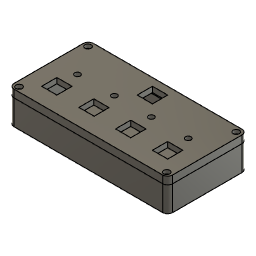
VFS5-fusion-file (Autodesk Fusion 360 design; units mm, degrees)
Autodesk Fusion 360 part; units mm, degrees
sketch "Plate" plane through (0, 0, 0) normal (0, 1, 0) x (1, 0, 0)
  line L0 (0, 0) -> (14, 0)
  line L1 (14, 0) -> (14, -14)
  line L2 (14, -14) -> (0, -14)
  line L3 (0, -14) -> (0, 0)
  line L4 (14, 0) -> (34, 0) construction
  line L5 (34, 0) -> (48, 0)
  line L6 (48, 0) -> (48, -13.6963)
  line L7 (48, -13.6963) -> (34, -13.6963)
  line L8 (34, -13.6963) -> (34, 0)
  line L9 (48, 0) -> (68, 0) construction
  line L10 (68, 0) -> (82, 0)
  line L11 (82, 0) -> (82, -14)
  line L12 (82, -14) -> (68, -14)
  line L13 (68, -14) -> (68, 0)
  line L14 (82, 0) -> (102, 0) construction
  line L15 (102, 0) -> (116, 0)
  line L16 (116, 0) -> (116, -14)
  line L17 (116, -14) -> (102, -14)
  line L18 (102, -14) -> (102, 0)
  line L19 (7, 0) -> (7, 12)
  circle A0 centre (7, 12) radius 2.55
  line L20 (41, 0) -> (41, 12)
  circle A1 centre (41, 12) radius 2.55
  line L21 (75, 0) -> (75, 12)
  circle A2 centre (75, 12) radius 2.55
  line L22 (109, 0) -> (109, 12)
  circle A3 centre (109, 12) radius 2.55
  line L23 (58, 0) -> (58, 30) construction
  line L24 (51, 23) -> (65, 23)
  line L25 (65, 23) -> (65, 37)
  line L26 (65, 37) -> (51, 37)
  line L27 (51, 37) -> (51, 23)
  line L28 (51, 23) -> (65, 37) construction
  line L29 (65, 23) -> (51, 37) construction
  line L30 (65, 37) -> (65, 42)
  line L31 (-5, -14) -> (-5, -19)
  line L32 (116, -19) -> (121, -19)
  line L33 (121, -19) -> (121, 42)
  line L34 (121, 42) -> (-5, 42)
  line L35 (-5, 42) -> (-5, -19)
  line L36 (-5, -19) -> (121, -19)
  line L37 (121, -19) -> (121, 42)
  line L38 (-5, 42) -> (-15, 42)
  line L39 (-15, 42) -> (-15, 44)
  line L40 (121, -29) -> (131, -29)
  line L41 (131, -29) -> (-15, -29)
  line L42 (-15, -29) -> (-15, 44)
  line L43 (-15, 44) -> (131, 44)
  line L44 (131, 44) -> (131, -29)
  point P0 (58, 30)
  dimension "d1" = 14
  dimension "d2" = 14
  dimension "d3" = 20
  dimension "d4" = 14
  dimension "d5" = 20
  dimension "d6" = 14
  dimension "d7" = 14
  dimension "d8" = 20
  dimension "d9" = 14
  dimension "d10" = 14
  dimension "d11" = 12
  dimension "d12" = 5.1
  dimension "d13" = 12
  dimension "d14" = 5.1
  dimension "d15" = 12
  dimension "d16" = 5.1
  dimension "d17" = 12
  dimension "d18" = 5.1
  dimension "d20" = 14
  dimension "d21" = 14
  dimension "d22" = 30
  dimension "d26" = 5
  dimension "d29" = 5
  dimension "d30" = 126
  dimension "d31" = 61
  constraint horizontal L0
  constraint vertical L1
  constraint horizontal L2
  constraint vertical L3
  constraint coincident L0.start L3.end
  constraint perpendicular L1 L4
  constraint horizontal L5
  constraint vertical L6
  constraint horizontal L7
  constraint vertical L8
  constraint perpendicular L6 L9
  constraint horizontal L10
  constraint vertical L11
  constraint horizontal L12
  constraint vertical L13
  constraint perpendicular L11 L14
  constraint horizontal L15
  constraint vertical L16
  constraint horizontal L17
  constraint vertical L18
  constraint midpoint L0 L19.start
  constraint perpendicular L0 L19
  constraint coincident L19.end A0.centre
  constraint coincident L20.end A1.centre
  constraint coincident L21.end A2.centre
  constraint coincident L22.end A3.centre
  constraint midpoint L9 L23.start
  constraint horizontal L24
  constraint perpendicular L24 L25
  constraint parallel L24 L26
  constraint parallel L25 L27
  constraint coincident L28 P0
  constraint coincident L29 P0
  constraint coincident P0 L23.end
  constraint perpendicular L26 L30
  constraint horizontal L34
  constraint vertical L35
  constraint horizontal L36
  constraint vertical L37
  constraint perpendicular L35 L38
  constraint perpendicular L38 L39
  constraint horizontal L41
  constraint vertical L42
  constraint horizontal L43
  constraint vertical L44
  measures "d1" distance of L0.start L0.end
  measures "d2" distance of L0.start L2.end
  measures "d3" distance of L0.end L4.end
  measures "d4" distance of L4.end L5.end
  measures "d5" distance of L5.end L9.end
  measures "d6" distance of L9.end L10.end
  measures "d7" distance of L9.end L12.end
  measures "d8" distance of L10.end L14.end
  measures "d9" distance of L14.end L15.end
  measures "d10" distance of L14.end L17.end
  measures "d11" distance of L19.start L19.end
  measures "d12" diameter of A0
  measures "d13" distance of L20.start L20.end
  measures "d14" diameter of A1
  measures "d15" distance of L21.start L21.end
  measures "d16" diameter of A2
  measures "d17" distance of L22.start L22.end
  measures "d18" diameter of A3
  measures "d20" distance of L25.end L26.end
  measures "d21" distance of L24.end L25.end
  measures "d22" distance of L23.start P0
  measures "d26" distance of L16.end L32.start
  measures "d29" distance of L32.start L32.end
  measures "d30" distance of L33.end L34.end
  measures "d31" distance of L31.end L34.end
extrude "Extrude1" add sketch "Plate" along normal blind 5 contours L31 L32 L33 L34 L35 L36 L37 makes body 1
ref_plane "WorkPlane1" through (7, 0, 7) normal (0, 1, 0) x (1, 0, 0)
sketch "Sketch2" plane through (7, 0, 7) normal (0, 1, 0) x (1, 0, 0)
  line L0 (40.7424, 48.8029) -> (110.7424, 48.8029)
  line L1 (110.7424, 48.8029) -> (110.7424, -1.1971)
  line L2 (110.7424, -1.1971) -> (40.7424, -1.1971)
  line L3 (40.7424, -1.1971) -> (40.7424, 48.8029)
  line L4 (110.7424, 48.8029) -> (106.7424, 48.8029)
  line L5 (106.7424, 48.8029) -> (76.7424, 48.8029)
  line L6 (76.7424, 48.8029) -> (76.7424, 39.6229)
  line L7 (76.7424, 39.6229) -> (110.7424, 39.6229)
  dimension "d39" = 70
  dimension "d40" = 50
  dimension "d43" = 4
  dimension "d44" = 30
  constraint horizontal L0
  constraint vertical L1
  constraint horizontal L2
  constraint vertical L3
  constraint perpendicular L1 L4
  constraint perpendicular L1 L5
  constraint perpendicular L0 L6
  constraint coincident L1 L7.end
  constraint perpendicular L1 L7
  measures "d39" distance of L0.start L0.end
  measures "d40" distance of L0.start L2.end
  measures "d43" distance of L0.end L4.end
  measures "d44" distance of L4.end L5.end
extrude "Extrude2" add sketch "Sketch2" along normal blind 2 separate body makes body 2
extrude "Extrude3" add sketch "Sketch2" along normal blind 13 contours L0 L1 L4 L5 L6 L7 bodies 2
move_body "Move1" bodies 2 to x (1, 0, 0) y (0, 1, 0) z (0, 0, 1) at (-10, -15, 0)
extrude "Extrude4" add sketch "Plate" along normal blind 5 contours L39 L40 L41 L42 L43 L44 bodies 1
extrude "Extrude5" add sketch "Plate" against normal blind 25 separate body contours L39 L40 L41 L42 L43 L44 makes body 3
sketch "Sketch3" plane through (0, -25, 0) normal (0, -1, 0) x (1, 0, 0)
  line L0 (121, 19) -> (121, -42)
  line L1 (121, -42) -> (-5, -42)
  line L2 (-5, -42) -> (-5, 19)
  line L3 (-5, 19) -> (121, 19)
  line L4 (-15, -44) -> (131, -44)
  line L5 (131, -44) -> (131, 29)
  line L6 (131, 29) -> (-15, 29)
  line L7 (-15, 29) -> (-15, -44)
  line L8 (-5, 19) -> (121, 19)
  line L9 (121, 19) -> (121, -42)
  line L10 (121, -42) -> (-5, -42)
  line L11 (-5, -42) -> (-5, 19)
  constraint horizontal L8
  constraint vertical L9
  constraint horizontal L10
  constraint vertical L11
  constraint coincident L0.end L1.start
  constraint coincident L2.end L3.start
extrude "Extrude6" add sketch "Sketch3" against normal blind 2 contours L0 L1 L2 L3 L8 L9 L10 L11 bodies 3
move_body "Move2" bodies 2 to x (1, 0, 0) y (0, 1, 0) z (0, 0, 1) at (0, -4, -1)
sketch "Sketch4" plane through (0, 0, -42.8029) normal (0, 0, -1) x (-1, 0, 0)
  line L0 (-107.7424, -19) -> (-37.7424, -19)
  line L1 (-37.7424, -19) -> (-37.7424, -17)
  line L2 (-37.7424, -17) -> (-73.7424, -17)
  line L3 (-73.7424, -17) -> (-73.7424, -6)
  line L4 (-73.7424, -6) -> (-107.7424, -6)
  line L5 (-107.7424, -6) -> (-107.7424, -19)
  line L6 (-107.7424, -6) -> (-73.7424, -6)
  line L7 (-73.7424, -6) -> (-73.7424, -17)
  line L8 (-73.7424, -17) -> (-107.7424, -17)
  line L9 (-107.7424, -17) -> (-107.7424, -6)
  constraint horizontal L6
  constraint vertical L7
  constraint horizontal L8
  constraint vertical L9
  constraint coincident L2.end L3.start
  constraint coincident L4.end L5.start
extrude "Extrude7" cut sketch "Sketch4" along normal blind 8 contours L3 L4 L5 L6 L7 L8 L9 bodies 3
sketch "Sketch5" plane through (0, -19, 0) normal (0, -1, 0) x (1, 0, 0)
  line L0 (107.7424, -42.8029) -> (107.7424, 7.1971)
  line L1 (107.7424, 7.1971) -> (37.7424, 7.1971)
  line L2 (37.7424, 7.1971) -> (37.7424, -42.8029)
  line L3 (37.7424, -42.8029) -> (107.7424, -42.8029)
  line L4 (37.7424, 7.1971) -> (39.7424, 7.1971)
  line L5 (37.7424, 5.1971) -> (37.7424, 7.1971)
  line L6 (107.7424, -42.8029) -> (105.7424, -42.8029)
  line L7 (107.7424, -40.8029) -> (107.7424, -42.8029)
  line L8 (105.7424, -40.8029) -> (39.7424, -40.8029)
  line L9 (39.7424, -40.8029) -> (39.7424, 5.1971)
  line L10 (39.7424, 5.1971) -> (105.7424, 5.1971)
  line L11 (105.7424, 5.1971) -> (105.7424, -40.8029)
  dimension "d55" = 2
  dimension "d56" = 2
  dimension "d57" = 2
  dimension "d58" = 2
  constraint horizontal L4
  constraint vertical L5
  constraint coincident L1.end L2.start
  constraint horizontal L6
  constraint vertical L7
  constraint coincident L0.start L3.end
  constraint horizontal L8
  constraint vertical L9
  constraint horizontal L10
  constraint vertical L11
  measures "d55" distance of L1.end L4.end
  measures "d56" distance of L1.end L5.start
  measures "d57" distance of L0.start L6.end
  measures "d58" distance of L0.start L7.start
extrude "Extrude8" add sketch "Sketch5" along normal blind 5 bodies 3
extrude "Extrude9" cut 1 faces at (96.4091, -13.3333, -42.8029) along direction (0, 0, 1) blind 2 on bodies 3 bodies 3
sketch "Sketch6" plane through (0, -19, 0) normal (0, 1, 0) x (-1, 0, 0)
  line L0 (-107.7424, -42) -> (-37.7424, -42)
  line L1 (-37.7424, -42) -> (-37.7424, 7.1971)
  line L2 (-37.7424, 7.1971) -> (-107.7424, 7.1971)
  line L3 (-107.7424, 7.1971) -> (-107.7424, -42)
  line L4 (-105.7424, 5.1971) -> (-39.7424, 5.1971)
  line L5 (-39.7424, 5.1971) -> (-39.7424, -40.8029)
  line L6 (-39.7424, -40.8029) -> (-105.7424, -40.8029)
  line L7 (-105.7424, -40.8029) -> (-105.7424, 5.1971)
  line L8 (-37.7424, 7.1971) -> (-107.7424, 7.1971)
  line L9 (-107.7424, 7.1971) -> (-107.7424, 10.1971)
  line L10 (-107.7424, 10.1971) -> (-37.7424, 10.1971)
  line L11 (-37.7424, 10.1971) -> (-37.7424, 7.1971)
  dimension "d63" = 3
  constraint horizontal L8
  constraint vertical L9
  constraint horizontal L10
  constraint vertical L11
  constraint coincident L1.end L2.start
  measures "d63" distance of L1.end L10.end
extrude "Extrude10" add sketch "Sketch6" against normal blind 5 contours L2 L8 L9 L10 L11 bodies 3
extrude "Extrude11" add sketch "Sketch6" along normal blind 2 contours L2 L8 L9 L10 L11 bodies 3
fillet "Fillet1" radius 4.5 8 edges at (-15, 2.5, -44) (-15, 2.5, 29) (131, 2.5, 29) (131, 2.5, -44) (-15, -12.5, -44) (-15, -12.5, 29) (131, -12.5, 29) (131, -12.5, -44) on bodies 1 3
sketch "Sketch7" plane through (0, 5, 0) normal (0, 1, 0) x (-1, 0, 0)
  arc A0 (-131, -39.5) -> (-126.5, -44) centre (-126.5, -39.5) ccw
  line L0 (-126.5, -44) -> (10.5, -44)
  arc A1 (10.5, -44) -> (15, -39.5) centre (10.5, -39.5) ccw
  line L1 (15, -39.5) -> (15, 24.5)
  arc A2 (15, 24.5) -> (10.5, 29) centre (10.5, 24.5) ccw
  line L2 (10.5, 29) -> (-126.5, 29)
  arc A3 (-126.5, 29) -> (-131, 24.5) centre (-126.5, 24.5) ccw
  line L3 (-131, 24.5) -> (-131, -39.5)
  line L4 (-51, -23) -> (-51, -37)
  line L5 (-51, -37) -> (-65, -37)
  line L6 (-65, -37) -> (-65, -23)
  line L7 (-65, -23) -> (-51, -23)
  circle A4 centre (-109, -12) radius 2.55
  line L8 (-116, 14) -> (-102, 14)
  line L9 (-102, 14) -> (-102, 0)
  line L10 (-102, 0) -> (-116, 0)
  line L11 (-116, 0) -> (-116, 14)
  circle A5 centre (-75, -12) radius 2.55
  line L12 (-82, 14) -> (-68, 14)
  line L13 (-68, 14) -> (-68, 0)
  line L14 (-68, 0) -> (-82, 0)
  line L15 (-82, 0) -> (-82, 14)
  circle A6 centre (-41, -12) radius 2.55
  line L16 (-48, 13.6963) -> (-34, 13.6963)
  line L17 (-34, 13.6963) -> (-34, 0)
  line L18 (-34, 0) -> (-48, 0)
  line L19 (-48, 0) -> (-48, 13.6963)
  circle A7 centre (-7, -12) radius 2.55
  line L20 (-14, 14) -> (0, 14)
  line L21 (0, 14) -> (0, 0)
  line L22 (0, 0) -> (-14, 0)
  line L23 (-14, 0) -> (-14, 14)
  circle A8 centre (-125.9937, 24.8023) radius 1.75
  circle A9 centre (-125.9937, 24.8023) radius 1.75
  circle A10 centre (-125.9937, 24.8023) radius 1.75
  circle A11 centre (-125.9937, -39.1977) radius 1.75
  line L24 (-48, 0) -> (-75, 0)
  circle A12 centre (10.0063, 24.8023) radius 1.75
  circle A13 centre (10.3846, -39.0945) radius 1.75
  circle A14 centre (10.0063, 24.8023) radius 2.85
  circle A15 centre (10.3846, -39.0945) radius 2.85
  circle A16 centre (-125.9937, -39.1977) radius 2.85
  circle A17 centre (-125.9937, 24.8023) radius 2.85
  dimension "d71" = 3.5
  dimension "d72" = 3.5
  dimension "d73" = 3.5
  dimension "d74" = 3.5
  dimension "d77" = 3.5
  dimension "d78" = 3.5
  dimension "d81" = 5.7
  dimension "d82" = 5.7
  dimension "d83" = 5.7
  dimension "d84" = 5.7
  constraint coincident L18.end L19.start
  constraint midpoint L14 L24.end
  constraint concentric A12 A14
  constraint concentric A13 A15
  constraint concentric A11 A16
  constraint concentric A10 A17
  measures "d71" diameter of A8
  measures "d72" diameter of A9
  measures "d73" diameter of A10
  measures "d74" diameter of A11
  measures "d77" diameter of A12
  measures "d78" diameter of A13
  measures "d81" diameter of A14
  measures "d82" diameter of A15
  measures "d83" diameter of A16
  measures "d84" diameter of A17
extrude "Extrude12" cut sketch "Sketch7" against normal blind 31 contours A8 A9 A10 | A11 | A12 | A13 bodies 1 3
extrude "Extrude13" cut sketch "Sketch7" against normal blind 3.5 contours A14 | A15 | A16 | A17 bodies 1
extrude "Extrude14" cut sketch "Sketch7" against normal blind 30 contours A14 | A15 | A16 | A17 bodies 3
ref_plane "WorkPlane2" through (0, -25, 0) normal (0, 1, 0) x (-1, 0, 0)
extrude "Extrude15" add sketch "Sketch7" against normal blind 8.5 contours A14 | A15 | A16 | A17 bodies 3
extrude "Extrude16" cut sketch "Sketch7" 2 faces at (-12.4725, 5, 24.5737) (-12.8573, 5, -39.2361) against normal blind 5 contours A16 | A17 on bodies 3 bodies 3
sketch "Sketch8" plane through (0, 0, 0) normal (0, -1, 0) x (1, 0, 0)
  circle A0 centre (-10.0063, 24.8023) radius 1.75
  circle A1 centre (125.9937, 24.8023) radius 1.75
  circle A2 centre (-10.3846, -39.0945) radius 1.75
  circle A3 centre (125.9937, -39.1977) radius 1.75
  arc A4 (126.5, -44) -> (131, -39.5) centre (126.5, -39.5) ccw
  line L0 (131, -39.5) -> (131, 24.5)
  arc A5 (131, 24.5) -> (126.5, 29) centre (126.5, 24.5) ccw
  line L1 (126.5, 29) -> (-10.5, 29)
  arc A6 (-10.5, 29) -> (-15, 24.5) centre (-10.5, 24.5) ccw
  line L2 (-15, 24.5) -> (-15, -39.5)
  arc A7 (-15, -39.5) -> (-10.5, -44) centre (-10.5, -39.5) ccw
  line L3 (-10.5, -44) -> (126.5, -44)
  line L4 (51, -37) -> (51, -23)
  line L5 (51, -23) -> (65, -23)
  line L6 (65, -23) -> (65, -37)
  line L7 (65, -37) -> (51, -37)
  circle A8 centre (109, -12) radius 2.55
  line L8 (102, 14) -> (116, 14)
  line L9 (116, 14) -> (116, 0)
  line L10 (116, 0) -> (102, 0)
  line L11 (102, 0) -> (102, 14)
  circle A9 centre (75, -12) radius 2.55
  line L12 (68, 14) -> (82, 14)
  line L13 (82, 14) -> (82, 0)
  line L14 (82, 0) -> (68, 0)
  line L15 (68, 0) -> (68, 14)
  circle A10 centre (41, -12) radius 2.55
  line L16 (34, 13.6963) -> (48, 13.6963)
  line L17 (48, 13.6963) -> (48, 0)
  line L18 (48, 0) -> (34, 0)
  line L19 (34, 0) -> (34, 13.6963)
  circle A11 centre (7, -12) radius 2.55
  line L20 (0, 14) -> (14, 14)
  line L21 (14, 14) -> (14, 0)
  line L22 (14, 0) -> (0, 0)
  line L23 (0, 0) -> (0, 14)
  arc A12 (130, 24.5) -> (126.5, 28) centre (126.5, 24.5) ccw
  line L24 (126.5, 28) -> (-10.5, 28)
  arc A13 (-10.5, 28) -> (-14, 24.5) centre (-10.5, 24.5) ccw
  line L25 (-14, 24.5) -> (-14, -39.5)
  arc A14 (-14, -39.5) -> (-10.5, -43) centre (-10.5, -39.5) ccw
  line L26 (-10.5, -43) -> (126.5, -43)
  arc A15 (126.5, -43) -> (130, -39.5) centre (126.5, -39.5) ccw
  line L27 (130, -39.5) -> (130, 24.5)
  dimension "d94" = -1
extrude "Extrude17" add sketch "Sketch8" along normal blind 2 contours A4 L0 A5 L1 A6 L2 A7 L3 bodies 1
sketch "Sketch9" plane through (0, 0, 0) normal (0, 1, 0) x (-1, 0, 0)
  circle A0 centre (10.0063, 24.8023) radius 1.75
  circle A1 centre (-125.9937, 24.8023) radius 1.75
  circle A2 centre (-125.9937, -39.1977) radius 1.75
  circle A3 centre (10.3846, -39.0945) radius 1.75
  arc A4 (-131, -39.5) -> (-126.5, -44) centre (-126.5, -39.5) ccw
  line L0 (-126.5, -44) -> (10.5, -44)
  arc A5 (10.5, -44) -> (15, -39.5) centre (10.5, -39.5) ccw
  line L1 (15, -39.5) -> (15, 24.5)
  arc A6 (15, 24.5) -> (10.5, 29) centre (10.5, 24.5) ccw
  line L2 (10.5, 29) -> (-126.5, 29)
  arc A7 (-126.5, 29) -> (-131, 24.5) centre (-126.5, 24.5) ccw
  line L3 (-131, 24.5) -> (-131, -39.5)
  line L4 (-121, -42) -> (-121, 19)
  line L5 (-121, 19) -> (5, 19)
  line L6 (5, 19) -> (5, -42)
  line L7 (5, -42) -> (-121, -42)
  line L8 (10.5, 27.85) -> (-126.5, 27.85)
  arc A8 (-126.5, 27.85) -> (-129.85, 24.5) centre (-126.5, 24.5) ccw
  line L9 (-129.85, 24.5) -> (-129.85, -39.5)
  arc A9 (-129.85, -39.5) -> (-126.5, -42.85) centre (-126.5, -39.5) ccw
  line L10 (-126.5, -42.85) -> (10.5, -42.85)
  arc A10 (10.5, -42.85) -> (13.85, -39.5) centre (10.5, -39.5) ccw
  line L11 (13.85, -39.5) -> (13.85, 24.5)
  arc A11 (13.85, 24.5) -> (10.5, 27.85) centre (10.5, 24.5) ccw
  dimension "d97" = -1.15
extrude "Extrude18" cut sketch "Sketch9" against normal blind 2 contours A4 L0 A5 L1 A6 L2 A7 L3 bodies 3
extrude "Extrude19" cut 1 faces at (61.0758, -18.3333, 7.1971) along direction (0, 0, 1) blind 0.2 on bodies 3 bodies 3
sketch "Sketch10" plane through (0, 0, -42) normal (0, 0, 1) x (1, 0, 0)
  line L0 (73.7424, -17) -> (73.7424, -6)
  line L1 (73.7424, -6) -> (107.7424, -6)
  line L2 (107.7424, -6) -> (107.7424, -17)
  line L3 (107.7424, -17) -> (73.7424, -17)
  line L4 (107.7424, -19) -> (107.7424, -23)
  line L5 (107.7424, -23) -> (121, -23)
  line L6 (121, -23) -> (121, 0)
  line L7 (121, 0) -> (-5, 0)
  line L8 (-5, 0) -> (-5, -23)
  line L9 (-5, -23) -> (37.7424, -23)
  line L10 (37.7424, -23) -> (37.7424, -19)
  line L11 (37.7424, -19) -> (107.7424, -19)
  line L12 (-5, 0) -> (37.7424, 0)
  line L13 (37.7424, 0) -> (37.7424, -23)
  line L14 (37.7424, -23) -> (-5, -23)
  line L15 (-5, -23) -> (-5, 0)
  line L16 (37.7424, 0) -> (73.7424, 0)
  line L17 (73.7424, 0) -> (73.7424, -6)
  line L18 (73.7424, -6) -> (37.7424, -6)
  line L19 (37.7424, -6) -> (37.7424, 0)
  line L20 (73.7424, -6) -> (121, -6)
  line L21 (121, -6) -> (121, 0)
  line L22 (121, 0) -> (73.7424, 0)
  line L23 (73.7424, 0) -> (73.7424, -6)
  constraint horizontal L12
  constraint vertical L13
  constraint horizontal L14
  constraint vertical L15
  constraint coincident L9.end L10.start
  constraint coincident L7.end L8.start
  constraint horizontal L16
  constraint vertical L17
  constraint horizontal L18
  constraint vertical L19
  constraint coincident L0.end L1.start
  constraint horizontal L20
  constraint vertical L21
  constraint horizontal L22
  constraint vertical L23
  constraint coincident L6.end L7.start
extrude "Extrude20" add sketch "Sketch10" along normal blind 2 separate body contours L1 L6 L7 L17 L20 L21 L22 L23 | L7 L13 L16 L17 L18 L19 L23 | L7 L8 L9 L10 L12 L13 L14 L15 L19 makes body 4
chamfer "Chamfer1" distance 2 angle 45 1 edges at (79.3712, -6, -40) on bodies 4
combine "Combine1" operation add target body 4 tool bodies 3
hidden bodies 2
named bodies: "plate", "platine", "base", "Base"
